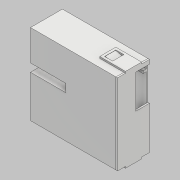
# Autodesk Inventor part: PhotogateCover
Saved by Autodesk Inventor 2018 (Build 220112000, 112)
## iProperties
Created: 2019-06-28
Part Number: PhotogateCover
Material: Generic
Document SubType Name: Modeling
Designer: mkivekas
Density: 1 g/cm^3
Appearance: Smooth - White
Author: mkivekas
Autodesk Inventor part; units mm, degrees
ref_plane "YZ Plane" through (0, 0, 0) normal (1, 0, 0) x (0, 1, 0)
sketch "Sketch1" plane through (0, 0, 0) normal (0, 1, 0) x (-1, 0, 0)
  line L0 (17.6061, 29.431) -> (-34.3939, 29.431)
  line L1 (-34.3939, -18.569) -> (17.6061, -18.569)
  line L2 (17.6061, -18.569) -> (17.6061, 5.431)
  line L3 (17.6061, 5.431) -> (-4.3939, 5.431)
  line L4 (-4.3939, 5.431) -> (-4.3939, 12.431)
  line L5 (-4.3939, 12.431) -> (17.6061, 12.431)
  line L6 (17.6061, 12.431) -> (17.6061, 29.431)
  line L7 (-34.3939, 29.431) -> (-34.3939, 30.431)
  line L8 (-34.3939, 30.431) -> (18.6061, 30.431)
  line L9 (18.6061, 30.431) -> (18.6061, 11.431)
  line L10 (18.6061, 11.431) -> (-3.3939, 11.431)
  line L11 (-3.3939, 11.431) -> (-3.3939, 6.431)
  line L12 (-3.3939, 6.431) -> (18.6061, 6.431)
  line L13 (18.6061, 6.431) -> (18.6061, -19.569)
  line L14 (-34.3939, -18.569) -> (-34.3939, -19.569)
  line L15 (-34.3939, -19.569) -> (18.6061, -19.569)
  point P0 (0, 0)
  dimension "d2" = 52
  dimension "d3" = 7
  dimension "d4" = 17
  dimension "d5" = 52
  dimension "d6" = 22
  dimension "d7" = 1
  dimension "d8" = 1
  dimension "d9" = 1
  dimension "d10" = 1
  dimension "d11" = 1
  dimension "d12" = 1
  dimension "d33" = 50
  constraints: 32 end point, 10 perpendicular, 3 point on line, 2 vertical, 1 horizontal, 1 parallel
  measures "d2" distance of L1.start L1.end
  measures "d3" distance of L3.end L4.end
  measures "d4" distance of L5.end L0.start
  measures "d5" distance of L0.start L0.end
  measures "d6" distance of L2.end L3.end
  measures "d7" distance between parallel lines of L15 L1
  measures "d8" distance between parallel lines of L13 L2
  measures "d9" distance between parallel lines of L0 L8
  measures "d10" distance between parallel lines of L3 L12
  measures "d11" distance between parallel lines of L5 L10
  measures "d12" distance between parallel lines of L4 L11
  measures "d33" distance between parallel lines of L8 L15
extrude "Extrusion1" add sketch "Sketch1" along normal blind 17.3
sketch "Sketch2" plane through (4.3939, 0, 5.431) normal (0, 0, -1) x (-1, 0, 0)
  line L0 (0, 17.3) -> (22, 17.3) projected
  line L1 (22, 0) -> (22, 17.3) projected
  point P0 (4.3939, 0)
  point P1 (13.9, 8.8)
  dimension "d15" = 8.5
  dimension "d16" = 8.1
  measures "d15" distance from line of L0 point (13.9, 8.8)
  measures "d16" distance from line of L1 point (13.9, 8.8)
hole "Hole1" at (-9.5061, 8.8, 5.431) direction (0, 0, 1) diameter 4 depth 8 tip angle 118
sketch "Sketch3" plane through (0, 17.3, 0) normal (0, 1, 0) x (1, 0, 0)
  line L0 (34.3939, -29.431) -> (34.3939, -30.431) projected
  line L1 (-18.6061, 19.569) -> (34.3939, 19.569) projected
  line L2 (34.3939, -30.431) -> (34.3939, 19.569)
  line L3 (34.3939, 19.569) -> (-18.6061, 19.569)
  line L4 (-18.6061, -6.431) -> (-18.6061, 19.569) projected
  line L5 (-18.6061, 19.569) -> (-18.6061, -6.431)
  line L6 (-18.6061, -6.431) -> (3.3939, -6.431)
  line L7 (3.3939, -6.431) -> (3.3939, -11.431) projected
  line L8 (3.3939, -6.431) -> (3.3939, -11.431)
  line L9 (3.3939, -11.431) -> (-18.6061, -11.431)
  line L10 (-18.6061, -11.431) -> (-18.6061, -30.431) projected
  line L11 (-18.6061, -11.431) -> (-18.6061, -30.431)
  line L12 (-18.6061, -30.431) -> (34.3939, -30.431) projected
  line L13 (-18.6061, -30.431) -> (34.3939, -30.431)
  point P0 (0, 0)
  constraints: 16 end point, 4 collinear, 3 perpendicular, 1 vertical
extrude "Extrusion2" add sketch "Sketch3" along normal blind 1
sketch "Sketch4" plane through (0, 17.3, 0) normal (0, -1, 0) x (1, 0, 0)
  line L0 (34.3939, 29.431) -> (34.3939, -18.569) projected
  line L1 (34.3939, -12.069) -> (-17.6, -12.069)
  line L2 (-17.6, -12.069) -> (-17.6, -10.569)
  line L3 (-17.6, -10.569) -> (34.3939, -10.569)
  line L4 (34.3939, -10.569) -> (34.3939, -12.069)
  line L5 (-17.6061, -18.569) -> (34.3939, -18.569) projected
  line L6 (34.3939, -13.619) -> (-17.6061, -13.619)
  line L7 (-17.6061, -13.619) -> (-17.6061, -15.619)
  line L8 (-17.6061, -15.619) -> (34.3939, -15.619)
  line L9 (34.3939, -15.619) -> (34.3939, -13.619)
  line L10 (34.3939, 23.831) -> (-17.6061, 23.831)
  line L11 (-17.6061, 23.831) -> (-17.6061, 25.331)
  line L12 (-17.6061, 25.331) -> (34.3939, 25.331)
  line L13 (34.3939, 25.331) -> (34.3939, 23.831)
  line L14 (34.3939, 26.881) -> (-17.6061, 26.881)
  line L15 (-17.6061, 26.881) -> (-17.6061, 29.431)
  line L16 (-17.6061, 29.431) -> (34.3939, 29.431)
  line L17 (34.3939, 29.431) -> (34.3939, 26.881)
  line L18 (-17.6061, 29.431) -> (34.3939, 29.431) projected
  line L19 (34.3939, 30.431) -> (-18.6061, 30.431) projected
  point P0 (0, 0)
  dimension "d26" = 6.5
  dimension "d27" = 1.5
  dimension "d28" = 2
  dimension "d29" = 1.55
  dimension "d30" = 1.5
  dimension "d31" = 4.1
  dimension "d32" = 1.55
  dimension "d47" = 1
  constraints: 32 end point, 8 parallel, 5 point on line, 4 horizontal, 4 perpendicular
  measures "d26" distance between parallel lines of L5 L1
  measures "d27" distance between parallel lines of L1 L3
  measures "d28" distance between parallel lines of L8 L6
  measures "d29" distance between parallel lines of L6 L1
  measures "d30" distance between parallel lines of L10 L12
  measures "d31" distance between parallel lines of L18 L12
  measures "d32" distance between parallel lines of L14 L12
  measures "d47" distance between parallel lines of L19 L16
extrude "Extrusion3" add sketch "Sketch4" along normal blind 2
sketch "Sketch5" plane through (0, 0, 0) normal (0, -1, 0) x (1, 0, 0)
  line L0 (-18.6061, -19.569) -> (-18.6061, 6.431) projected
  line L1 (34.3939, -19.569) -> (-18.6061, -19.569) projected
  line L2 (-18.6061, -19.569) -> (34.3939, -19.569)
  line L3 (34.3939, 29.431) -> (34.3939, 30.431) projected
  line L4 (34.3939, -19.569) -> (34.3939, 30.431)
  line L5 (-18.6061, 11.431) -> (-18.6061, 30.431) projected
  line L6 (34.3939, 30.431) -> (-18.6061, 30.431)
  line L7 (-18.6061, 30.431) -> (-18.6061, 11.431)
  line L8 (3.3939, 11.431) -> (3.3939, 6.431) projected
  line L9 (-18.6061, 11.431) -> (3.3939, 11.431)
  line L10 (3.3939, 11.431) -> (3.3939, 6.431)
  line L11 (3.3939, 6.431) -> (-18.6061, 6.431) projected
  line L12 (3.3939, 6.431) -> (-18.6061, 6.431)
  line L13 (-18.6061, 6.431) -> (-18.6061, -19.569)
  point P0 (0, 0)
  constraints: 16 end point, 5 perpendicular, 2 collinear, 1 horizontal
extrude "Extrusion4" add sketch "Sketch5" along normal blind 1.5
sketch "Sketch6" plane through (0, 0, 0) normal (0, 1, 0) x (1, 0, 0)
  line L0 (-17.6061, -29.431) -> (34.3939, -29.431) projected
  line L1 (-17.6061, -12.431) -> (-17.6061, -29.431) projected
  line L2 (34.3939, -29.431) -> (-17.6061, -29.431)
  line L3 (-17.6061, -29.431) -> (-17.6061, -26.881)
  line L4 (-17.6061, -26.881) -> (34.3939, -26.881)
  line L5 (34.3939, -26.881) -> (34.3939, -29.431)
  line L6 (34.3939, 18.569) -> (34.3939, -29.431) projected
  line L7 (34.3939, -25.331) -> (-17.6061, -25.331)
  line L8 (-17.6061, -25.331) -> (-17.6061, -23.831)
  line L9 (-17.6061, -23.831) -> (34.3939, -23.831)
  line L10 (34.3939, -23.831) -> (34.3939, -25.331)
  line L11 (-17.6061, 18.569) -> (-17.6061, -5.431) projected
  line L12 (34.3939, 10.569) -> (-17.6061, 10.569)
  line L13 (-17.6061, 10.569) -> (-17.6061, 12.069)
  line L14 (-17.6061, 12.069) -> (34.3939, 12.069)
  line L15 (34.3939, 12.069) -> (34.3939, 10.569)
  line L16 (34.3939, 13.619) -> (-17.6061, 13.619)
  line L17 (-17.6061, 13.619) -> (-17.6061, 15.619)
  line L18 (-17.6061, 15.619) -> (34.3939, 15.619)
  line L19 (34.3939, 15.619) -> (34.3939, 13.619)
  line L20 (34.3939, 18.569) -> (-17.6061, 18.569) projected
  point P0 (0, 0)
  dimension "d38" = 1.5
  dimension "d39" = 2
  dimension "d40" = 1.55
  dimension "d41" = 8
  dimension "d42" = 1.5
  dimension "d43" = 1.55
  dimension "d44" = 5.6
  constraints: 32 end point, 8 parallel, 7 point on line, 4 horizontal, 4 perpendicular
  measures "d38" distance between parallel lines of L14 L12
  measures "d39" distance between parallel lines of L18 L16
  measures "d40" distance between parallel lines of L16 L14
  measures "d41" distance between parallel lines of L20 L12
  measures "d42" distance between parallel lines of L9 L7
  measures "d43" distance between parallel lines of L7 L4
  measures "d44" distance from line of L0.end L9
extrude "Extrusion5" add sketch "Sketch6" along normal blind 2 contours L1 L4 L5 L0 | L1 L9 L6 L7 | L6 L16 L11 L18 | L6 L12 L11 L14
sketch "Sketch7" plane through (34.3939, 18.3, 30.431) normal (1, 0, 0) x (0, 0, -1)
  line L0 (0, 0) -> (0, -19.8) projected
  line L1 (50, 0) -> (24, 0) projected
  line L2 (0, -19.8) -> (50, -19.8)
  line L3 (50, -19.8) -> (50, 0)
  line L4 (50, 0) -> (0, 0)
  line L5 (0, 0) -> (0, -19.8)
  point P0 (30.431, -18.3)
  constraints: 8 end point, 2 parallel, 1 horizontal, 1 perpendicular
extrude "Extrusion6" add sketch "Sketch7" along normal blind 1 separate body
sketch "Sketch8" plane through (35.3939, 18.3, 30.431) normal (1, 0, 0) x (0, 0, -1)
  line L0 (50, 0) -> (0, 0) projected
  line L1 (2.55, 0) -> (23.55, 0)
  line L2 (23.55, 0) -> (23.55, -8.5)
  line L3 (23.55, -8.5) -> (2.55, -8.5)
  line L4 (2.55, -8.5) -> (2.55, 0)
  line L5 (0, 0) -> (0, -19.8) projected
  point P0 (30.431, -18.3)
  dimension "d50" = 2.55
  dimension "d51" = 21
  dimension "d52" = 8.5
  constraints: 8 end point, 2 parallel, 1 horizontal, 1 perpendicular, 1 point on line
  measures "d50" distance between parallel lines of L5 L4
  measures "d51" distance of L2.end L3.end
  measures "d52" distance of L3.end L1.start
extrude "Extrusion7" cut sketch "Sketch8" against normal blind 1.1 bodies 2
sketch "Sketch9" plane through (34.3939, -1.5, 30.431) normal (0, 0, 1) x (1, 0, 0)
  line L0 (0, 0) -> (0, 19.8) projected
  line L1 (1, 0) -> (1, 19.8) projected
  line L2 (0, 0) -> (1, 19.8)
  line L3 (0, 19.8) -> (1, 19.8) projected
  line L4 (1, 19.8) -> (0, 19.8)
  line L5 (0, 19.8) -> (1, 0)
  line L6 (0, 0) -> (1, 0) projected
  line L7 (1, 0) -> (0, 0)
  line L8 (1, 14.9) -> (0, 14.9)
  line L9 (0, 14.9) -> (0, 4.9)
  line L10 (0, 4.9) -> (1, 4.9)
  line L11 (1, 4.9) -> (1, 14.9)
  line L12 (1, 14.9) -> (0, 4.9) construction
  line L13 (0, 14.9) -> (1, 4.9) construction
  line L14 (0, 4.9) -> (-15, 4.9)
  line L15 (-15, 4.9) -> (-15, 14.9)
  line L16 (-15, 14.9) -> (0, 14.9)
  line L17 (0, 14.9) -> (0, 4.9)
  point P0 (-34.3939, 1.5)
  point P1 (0.5, 9.9)
  dimension "d55" = 10
  dimension "d56" = 15
  constraints: 28 end point, 5 equal length, 3 midpoint, 2 horizontal, 2 perpendicular, 1 point on line
  measures "d55" distance between parallel lines of L8 L10
  measures "d56" distance between parallel lines of L0 L15
extrude "Extrusion8" add sketch "Sketch9" along normal blind 1 contours L14 L15 L16 L0 | L0 L8 L5 L2 L10 | L2 L5 L10 | L5 L8 L2 | L2 L8 L1 L10 L5 bodies 2
sketch "Sketch10" plane through (34.3939, -1.5, -19.569) normal (0, 0, -1) x (-1, 0, 0)
  line L0 (0, 19.8) -> (-1, 19.8) projected
  line L1 (-1, 4.9) -> (-1, 0) projected
  line L2 (0, 19.8) -> (-1, 0)
  line L3 (0, 0) -> (-1, 0) projected
  line L4 (-1, 0) -> (0, 0)
  line L5 (-1, 19.8) -> (-1, 14.9) projected
  line L6 (0, 0) -> (-1, 19.8)
  line L7 (0, 14.9) -> (0, 4.9) projected
  line L8 (-1, 14.9) -> (0, 14.9)
  line L9 (0, 14.9) -> (0, 4.9)
  line L10 (0, 4.9) -> (-1, 4.9)
  line L11 (-1, 4.9) -> (-1, 14.9)
  line L12 (-1, 14.9) -> (0, 4.9) construction
  line L13 (0, 14.9) -> (-1, 4.9) construction
  line L14 (15, 4.9) -> (0, 4.9) projected
  line L15 (0, 14.9) -> (15, 14.9)
  line L16 (15, 14.9) -> (15, 4.9)
  line L17 (15, 4.9) -> (0, 4.9)
  line L18 (0, 4.9) -> (0, 14.9)
  point P0 (34.3939, 1.5)
  point P1 (-0.5, 9.9)
  constraints: 26 end point, 5 equal length, 3 midpoint, 2 horizontal, 2 perpendicular
extrude "Extrusion9" add sketch "Sketch10" along normal blind 1 contours L8 L7 L10 L6 L2 | L2 L6 L8 | L8 L6 L2 L10 L11 | L6 L10 L2 | L15 L16 L14 L7 bodies 2
sketch "Sketch11" plane through (34.3939, -1.5, -20.569) normal (0, 0, -1) x (-1, 0, 0)
  line L0 (13.5, 13.4) -> (8.5, 13.4)
  line L1 (8.5, 13.4) -> (8.5, 6.4)
  line L2 (8.5, 6.4) -> (13.5, 6.4)
  line L3 (13.5, 6.4) -> (13.5, 13.4)
  line L4 (15, 4.9) -> (15, 14.9) projected
  line L5 (15, 14.9) -> (-1, 14.9) projected
  line L6 (-1, 4.9) -> (15, 4.9) projected
  point P0 (34.3939, 1.5)
  dimension "d61" = 1.5
  dimension "d62" = 1.5
  dimension "d63" = 1.5
  dimension "d64" = 5
  constraints: 8 end point, 2 parallel, 1 horizontal, 1 perpendicular
  measures "d61" distance between parallel lines of L4 L3
  measures "d62" distance between parallel lines of L5 L0
  measures "d63" distance between parallel lines of L6 L2
  measures "d64" distance between parallel lines of L1 L3
extrude "Extrusion10" cut sketch "Sketch11" against normal blind 100 bodies 2
sketch "Sketch12" plane through (34.3939, 18.3, -19.569) normal (0, 0, -1) x (-1, 0, 0)
  line L0 (13.4, -6.7) -> (8.6, -6.7)
  line L1 (8.6, -6.7) -> (8.6, -13.1)
  line L2 (8.6, -13.1) -> (13.4, -13.1)
  line L3 (13.4, -13.1) -> (13.4, -6.7)
  line L4 (13.5, -6.4) -> (13.5, -13.4) projected
  line L5 (13.5, -13.4) -> (8.5, -13.4) projected
  line L6 (8.5, -6.4) -> (13.5, -6.4) projected
  line L7 (8.5, -13.4) -> (8.5, -6.4) projected
  point P0 (34.3939, -18.3)
  dimension "d67" = 0.1
  dimension "d68" = 0.3
  dimension "d69" = 0.3
  dimension "d70" = 0.1
  constraints: 8 end point, 2 parallel, 1 horizontal, 1 perpendicular
  measures "d67" distance between parallel lines of L4 L3
  measures "d68" distance between parallel lines of L5 L2
  measures "d69" distance between parallel lines of L6 L0
  measures "d70" distance between parallel lines of L7 L1
extrude "Extrusion11" add sketch "Sketch12" along normal blind 1 contours L3 L2 L1 L0 bodies 1
ref_plane "Work Plane2" through (20.9939, 11.6, -20.569) normal (0.2039543, 0, -0.9789804) x (0.9789804, 0, 0.2039543)
split_face "Split1"
sketch "Sketch13" plane through (20.9939, 11.6, -20.569) normal (0.2039543, 0, -0.9789804) x (0.9789804, 0, 0.2039543)
  line L0 (4.9031, 6.4) -> (4.9031, 0) projected
  line L1 (0.204, 6.4) -> (0, 6.4) projected
  line L2 (4.9031, 0) -> (0, 0)
  line L3 (0, 0) -> (0, 6.4)
  line L4 (0, 6.4) -> (4.9031, 6.4)
  line L5 (4.9031, 6.4) -> (4.9031, 0)
  point P0 (-16.3575, 11.6)
  constraints: 8 end point, 2 parallel, 1 horizontal, 1 perpendicular
extrude "Extrusion12" cut sketch "Sketch13" along normal blind 2 bodies 1
sketch "Sketch14" plane through (-18.6061, 18.3, 30.431) normal (0, 0, 1) x (1, 0, 0)
  line L0 (39.6, -13.1) -> (44.4, -13.1) projected
  line L1 (44.4, -6.7) -> (39.6, -6.7) projected
  line L2 (39.6, -13.1) -> (44.4, -13.1)
  line L3 (44.4, -13.1) -> (44.4, -6.7)
  line L4 (44.4, -6.7) -> (39.6, -6.7)
  line L5 (39.6, -6.7) -> (39.6, -13.1)
  point P0 (18.6061, -18.3)
  constraints: 8 end point, 2 parallel, 1 horizontal, 1 perpendicular
extrude "Extrusion13" add sketch "Sketch14" along normal blind 1 bodies 1
ref_plane "Work Plane3" through (20.9939, 11.6, 31.431) normal (-0.2039543, 0, -0.9789804) x (0.9789804, 0, -0.2039543)
sketch "Sketch15" plane through (20.9939, 11.6, 31.431) normal (-0.2039543, 0, -0.9789804) x (0.9789804, 0, -0.2039543)
  line L0 (4.9031, 6.4) -> (0.204, 6.4) projected
  line L1 (4.6991, 0) -> (0, 0) projected
  line L2 (4.9031, 6.4) -> (0, 6.4)
  line L3 (0, 6.4) -> (0, 0)
  line L4 (0, 0) -> (4.9031, 0)
  line L5 (4.9031, 0) -> (4.9031, 6.4)
  point P0 (-14.1421, 11.6)
  constraints: 8 end point, 2 parallel, 1 horizontal, 1 perpendicular
extrude "Extrusion14" cut sketch "Sketch15" against normal blind 1 bodies 1
body "Solid1"
body "Solid2"
